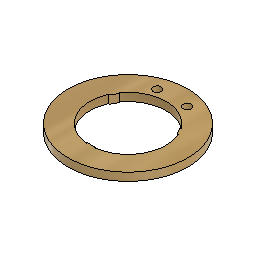
SPACER_UPPER (Autodesk Fusion 360 design; units mm, degrees)
Autodesk Fusion 360 part; units mm, degrees
sketch "Sketch1" plane through (0, 0, 0) normal (0, 0, 1) x (1, 0, 0)
  circle A0 centre (0, 0) radius 29.75
  circle A1 centre (0, 0) radius 18.925
  line L0 (0, 0) -> (0, 29.75) construction
  circle A2 centre (-7.5, 22) radius 2
  circle A3 centre (7.5, 22) radius 2
  line L1 (0, -18.419) -> (2, -18.419)
  line L2 (2, -18.419) -> (2, -18.819)
  line L3 (0, -18.925) -> (0, -18.419) construction
  line L4 (-2, -18.419) -> (-2, -18.819)
  line L5 (0, -18.419) -> (-2, -18.419)
  line L6 (16.9513, 7.4775) -> (17.2978, 7.6775)
  line L7 (15.9513, 9.2095) -> (16.9513, 7.4775)
  line L8 (15.9513, 9.2095) -> (14.9513, 10.9416)
  line L9 (14.9513, 10.9416) -> (15.2978, 11.1416)
  line L10 (-14.9513, 10.9416) -> (-15.2978, 11.1416)
  line L11 (-15.9513, 9.2095) -> (-14.9513, 10.9416)
  line L12 (-15.9513, 9.2095) -> (-16.9513, 7.4775)
  line L13 (-16.9513, 7.4775) -> (-17.2978, 7.6775)
  dimension "d1" = 59.5
  dimension "d78" = 37.85
  dimension "d131" = 4
  dimension "d132" = 7.5
  dimension "d135" = 2
  dimension "d136" = 0.4
  dimension "d138" = 360
  constraint coincident A0.centre A1.centre
  constraint coincident A0 L0.end
  constraint vertical L0
  constraint symmetric L0 A2 A3
  constraint horizontal L1
  constraint vertical L2
  constraint vertical L3
  constraint coincident A1 L2.end
  constraint coincident A1 L3.start
  constraint symmetric L1.start L3 L5.start
  constraint symmetric L1.end L3 L4.start
  constraint symmetric L3 L2.end L4.end
  measures "d1" diameter of A0
  measures "d78" diameter of A1
  measures "d131" diameter of A2
  measures "d132" distance of L0 A2.centre
  measures "d135" distance of L1.start L1.end
  measures "d136" distance of L1.end L2.end
extrude "Extrude16" add sketch "Sketch1" along normal blind 4 contours A0 | A1 L6 L7 L8 L9 | A1 L1 L2 L4 L5 | A1 L10 L11 L12 L13 | A2 | A3
extrude "Extrude17" cut sketch "Sketch1" along normal blind 4 contours A2 | A3
